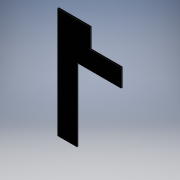
# Autodesk Inventor part: BA03
Saved by Autodesk Inventor 2017 (Build 210142000, 142)
## iProperties
Created: 2018-10-18
Part Number: BA03
Material: ABS Plastic
Document SubType Name: Modeling
Designer: Dell
Density: 1.06 g/cm^3
Appearance: Smooth - Black
Author: Dell
Autodesk Inventor part; units mm, degrees
ref_plane "YZ Plane" through (0, 0, 0) normal (1, 0, 0) x (0, 1, 0)
ref_plane "XZ Plane" through (0, 0, 0) normal (0, 1, 0) x (-1, 0, 0)
ref_plane "XY Plane" through (0, 0, 0) normal (0, 0, 1) x (1, 0, 0)
sketch "Sketch1" plane through (0, 0, 0) normal (0, 0, 1) x (1, 0, 0)
  line L0 (0, 0) -> (307.2255, 0)
  line L1 (307.2255, 0) -> (307.2255, -177.8)
  line L2 (307.2255, -177.8) -> (0, -177.8)
  line L3 (0, -177.8) -> (0, 0)
  line L4 (460.8382, 266.0651) -> (307.2255, 0)
  line L5 (307.2255, 0) -> (0, 0)
  line L6 (0, 0) -> (-153.6127, 266.0651)
  line L7 (-153.6127, 266.0651) -> (0, 532.1302)
  line L8 (0, 532.1302) -> (307.2255, 532.1302)
  line L9 (307.2255, 532.1302) -> (460.8382, 266.0651)
  point P0 (153.6127, 266.0651)
  dimension "d1" = 177.8
  dimension "d39" = 307.2255
  constraints: 20 end point, 2 parallel, 1 horizontal, 1 perpendicular, 13 other
  measures "d1" distance of L0.end L1.end
  measures "d39" distance of L0.start L0.end
extrude "Extrusion1" add sketch "Sketch1" along normal blind 6.35 contours L0 L1 L2 L3
sketch "Sketch2" plane through (0, 0, 0) normal (0, 1, 0) x (1, 0, 0)
  line L0 (307.2255, -6.35) -> (0, -6.35) projected
  line L1 (0, -6.35) -> (-3.6662, -6.35)
  line L2 (-3.6662, -6.35) -> (0, 0)
  line L3 (0, 0) -> (0, -6.35) projected
  line L4 (0, 0) -> (0, -6.35) projected
  line L5 (0, -6.35) -> (0, 0)
  line L6 (307.2255, -6.35) -> (310.8917, -6.35)
  line L7 (307.2255, 0) -> (307.2255, -6.35) projected
  line L8 (310.8917, -6.35) -> (307.2255, 0)
  line L9 (307.2255, 0) -> (307.2255, -6.35)
  dimension "d4" = 30
  dimension "d5" = 60
  constraints: 12 end point, 2 collinear, 2 horizontal
  measures "d4" angle of L3 L2
  measures "d5" angle of L6 L8
extrude "Extrusion2" add sketch "Sketch2" against normal blind 177.8
sketch "Sketch3" plane through (0, 0, 6.35) normal (0, 0, 1) x (1, 0, 0)
  line L0 (81.3338, -88.9) -> (281.3338, -88.9)
  line L1 (281.3338, -88.9) -> (281.3338, 0)
  line L2 (281.3338, 0) -> (81.3338, 0)
  line L3 (81.3338, 0) -> (81.3338, -88.9)
  line L4 (-3.6662, 0) -> (310.8917, 0) projected
  line L5 (81.3338, -88.9) -> (192.81, -88.9)
  line L6 (121.05, 0) -> (81.3338, 0)
  line L7 (81.3338, 0) -> (81.3338, -88.9)
  line L8 (281.3338, 0) -> (169.304, 0)
  line L9 (156.3338, -88.9) -> (281.3338, -88.9)
  line L10 (281.3338, -88.9) -> (281.3338, 0)
  line L11 (81.3338, 0) -> (156.3338, 0)
  line L12 (156.3338, 0) -> (156.3338, -88.9)
  line L13 (156.3338, -88.9) -> (81.3338, -88.9)
  line L14 (81.3338, -88.9) -> (81.3338, 0)
  line L15 (281.3338, 0) -> (281.3338, -88.9)
  line L16 (281.3338, -88.9) -> (281.3338, 0)
  line L17 (-3.6662, 0) -> (-3.6662, -177.8) projected
  point P0 (0, 0)
  point P1 (281.3338, -44.45)
  point P2 (153.6127, 0)
  point P3 (153.6127, 0)
  dimension "d8" = 200
  dimension "d9" = 88.9
  dimension "d14" = 75
  dimension "d33" = 85
  constraints: 32 end point, 6 parallel, 5 midpoint, 4 horizontal, 4 point on line, 2 coincident, 2 perpendicular, 2 vertical, 1 collinear, 4 other
  measures "d8" distance of L1.end L2.end
  measures "d9" distance of L0.end L1.end
  measures "d14" distance between parallel lines of L3 L12
  measures "d33" distance between parallel lines of L17 L14
extrude "Extrusion3" cut sketch "Sketch3" against normal through all contours L12 L2 L1 L0
sketch "Sketch5" plane through (0, 0, 6.35) normal (0, 0, 1) x (1, 0, 0)
  line L0 (310.8917, -177.8) -> (-3.6662, -177.8) projected
  line L1 (-3.6662, -177.8) -> (91.5838, -177.8)
  line L2 (91.5838, -177.8) -> (91.5838, -533.4)
  line L3 (91.5838, -533.4) -> (-3.6662, -533.4)
  line L4 (-3.6662, -533.4) -> (-3.6662, -177.8)
  point P0 (0, 0)
  dimension "d23" = 95.25
  dimension "d24" = 355.6
  constraints: 8 end point, 2 parallel, 1 horizontal, 1 perpendicular
  measures "d23" distance between parallel lines of L2 L4
  measures "d24" distance of L3.end L0.end
extrude "Extrusion5" add sketch "Sketch5" against normal blind 10
sketch "Sketch6" plane through (-3.6662, -177.8, -3.65) normal (0, 1, 0) x (1, 0, 0)
  line L0 (0, -10) -> (3.6662, -3.65) projected
  line L1 (0, 0) -> (95.25, 0) projected
  line L2 (0, -10) -> (0, 0) projected
  line L3 (95.25, -3.65) -> (3.6662, -3.65) projected
  line L4 (95.25, -3.65) -> (95.25, 0) projected
  point P0 (3.6662, -3.65)
extrude "Extrusion6" cut sketch "Sketch6" against normal through all
sketch "Sketch9" plane through (0, 0, 6.35) normal (0, 0, 1) x (1, 0, 0)
  line L0 (281.3338, -88.9) -> (156.3338, -88.9) projected
  line L1 (310.8917, 0) -> (310.8917, -177.8) projected
  line L2 (281.3338, -88.9) -> (310.8917, -88.9)
  line L3 (310.8917, -88.9) -> (310.8917, 0)
  line L4 (310.8917, 0) -> (281.3338, 0)
  line L5 (281.3338, 0) -> (281.3338, -88.9)
  point P0 (0, 0)
  constraints: 8 end point, 2 parallel, 1 horizontal, 1 perpendicular
extrude "Extrusion8" cut sketch "Sketch9" against normal through all
sketch "Sketch10" plane through (0, 0, 0) normal (0, 1, 0) x (1, 0, 0)
  line L0 (0, 0) -> (0, -6.35)
  line L1 (-3.6662, -6.35) -> (156.3338, -6.35) projected
  line L2 (0, -6.35) -> (-3.6662, -6.35)
  line L3 (0, 0) -> (-3.6662, -6.35) projected
  line L4 (0, 0) -> (-3.6662, -6.35)
  line L5 (0, 0) -> (156.3338, 0) projected
  line L6 (-3.6662, -6.35) -> (0, 0)
  line L7 (156.3338, 0) -> (307.2255, 0) projected
  line L8 (307.2255, 0) -> (307.2255, -6.35)
  line L9 (310.8917, -6.35) -> (156.3338, -6.35) projected
  line L10 (307.2255, -6.35) -> (310.8917, -6.35)
  line L11 (307.2255, 0) -> (310.8917, -6.35) projected
  line L12 (310.8917, -6.35) -> (307.2255, 0)
  line L13 (307.2255, 0) -> (310.8917, -6.35)
  constraints: 16 end point, 5 collinear, 2 vertical, 1 perpendicular, 1 point on line
extrude "Extrusion9" cut sketch "Sketch10" against normal through all contours L0 L1 L3 | L11 L9 L8
sketch "Sketch11" plane through (0, 0, 6.35) normal (0, 0, 1) x (1, 0, 0)
  line L0 (0, 0) -> (-3.6662, 0)
  line L1 (-3.6662, 0) -> (-3.6662, -533.4)
  line L2 (-3.6662, -533.4) -> (0, -533.4)
  line L3 (0, -533.4) -> (0, 0)
  line L4 (91.5838, -177.8) -> (91.5838, -533.4) projected
  dimension "d40" = 95.25
  constraints: 8 end point, 2 parallel, 1 coincident, 1 horizontal, 1 perpendicular
  measures "d40" distance between parallel lines of L4 L1
extrude "Extrusion10" add sketch "Sketch11" against normal blind 6.35
sketch "Sketch12" plane through (0, 0, 6.35) normal (0, 0, 1) x (1, 0, 0)
  line L0 (-3.6662, 0) -> (156.3338, 0) projected
  line L1 (156.3338, 0) -> (-3.6662, 0)
  line L2 (-3.6662, 0) -> (-3.6662, 6.35)
  line L3 (-3.6662, 6.35) -> (156.3338, 6.35)
  line L4 (156.3338, 6.35) -> (156.3338, 0)
  point P0 (0, 0)
  point P1 (-3.6662, 3.175)
  dimension "d43" = 6.35
  constraints: 8 end point, 2 parallel, 1 horizontal, 1 midpoint, 1 perpendicular, 1 vertical alignment
  measures "d43" distance between parallel lines of L0 L3
extrude "Extrusion11" add sketch "Sketch12" against normal blind 6.35
body "Solid1"
